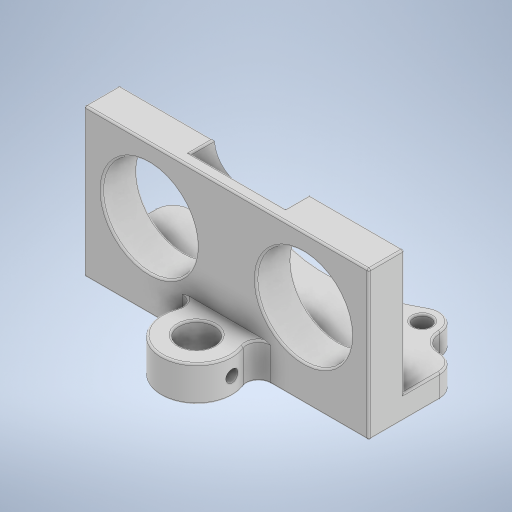
# Autodesk Inventor part: Front Sensor Mount
Saved by Autodesk Inventor 2023 (Build 270158000, 158)
## iProperties
Created: 2023-11-02
Part Number: Front Sensor Mount
Material: Generic
Document SubType Name: Modeling
Designer: Eric
Density: 1 g/cm^3
Appearance: Default
Author: Eric
Autodesk Inventor part; units mm, degrees
ref_plane "YZ Plane" through (0, 0, 0) normal (1, 0, 0) x (0, 1, 0)
ref_plane "XZ Plane" through (0, 0, 0) normal (0, 1, 0) x (-1, 0, 0)
ref_plane "XY Plane" through (0, 0, 0) normal (0, 0, 1) x (1, 0, 0)
sketch "Sketch1" plane through (0, 0, 0) normal (0, 1, 0) x (-1, 0, 0)
  circle A0 centre (15, -5) radius 1.45
  circle A1 centre (-15, -5) radius 1.45
  arc A2 (13.5033, -7.6) -> (18, -5) centre (15, -5) ccw
  arc A3 (-18, -5) -> (-13.5033, -7.6) centre (-15, -5) ccw
  arc A4 (13.5033, -7.6) -> (-13.5033, -7.6) centre (0, -31.058) ccw
  line L0 (24, 1) -> (24, 13)
  line L1 (-24, 1) -> (-24, 13)
  arc A5 (21, -2) -> (24, 1) centre (21, 1) ccw
  arc A6 (21, -2) -> (18, -5) centre (21, -5) ccw
  line L2 (0, -11.9168) -> (0, 19.826) construction
  arc A7 (-24, 1) -> (-21, -2) centre (-21, 1) ccw
  arc A8 (-18, -5) -> (-21, -2) centre (-21, -5) ccw
  circle A9 centre (0, 18) radius 3
  arc A10 (5.5621, 15.75) -> (-5.5621, 15.75) centre (0, 18) ccw
  line L3 (24, 13) -> (7.4162, 13)
  line L4 (-7.4162, 13) -> (-24, 13)
  arc A11 (5.5621, 15.75) -> (7.4162, 13) centre (7.4162, 15) ccw
  arc A12 (-7.4162, 13) -> (-5.5621, 15.75) centre (-7.4162, 15) ccw
  point P0 (0, 0)
  point P1 (0, 13)
  point P2 (3.3166, 13)
  point P3 (-3.3166, 13)
  dimension "d0" = 2.9
  dimension "d1" = 30
  dimension "d3" = 3
  dimension "d6" = 5
  dimension "d8" = 2.6
  dimension "d10" = 18
  dimension "d11" = 12
  dimension "d12" = 6
  dimension "d14" = 6
  dimension "d15" = 48
  dimension "d16" = 5
  dimension "d17" = 2
  constraints: 22 point on circle, 13 centre point, 12 end point, 9 tangent, 4 equal radius, 4 horizontal alignment, 4 symmetric about line, 3 concentric, 3 point on line, 3 vertical, 2 horizontal, 2 vertical alignment, 1 collinear, 2 other
  measures "d0" diameter of A0
  measures "d1" distance of A1.centre A0.centre
  measures "d3" radius of A2
  measures "d6" vertical distance of point (0, 0) A0.centre
  measures "d8" vertical distance of A0.centre A2.start
  measures "d10" vertical distance of A0.centre L0.end
  measures "d11" distance of L0.start L0.end
  measures "d12" diameter of A9
  measures "d14" radius of A10
  measures "d15" distance between parallel lines of L1 L0
  measures "d16" distance from line of L4 A9.centre
  measures "d17" radius of A11
extrude "Extrusion1" add sketch "Sketch1" along normal blind 4
sketch "Sketch3" plane through (0, 4, 0) normal (0, 1, 0) x (1, 0, 0)
  line L0 (-24, -13) -> (-7.4162, -13) projected
  line L1 (24, -13) -> (24, -1) projected
  line L2 (-24, -13) -> (24, -13)
  line L3 (24, -13) -> (24, -7)
  line L4 (24, -7) -> (-24, -7)
  line L5 (-24, -7) -> (-24, -13)
  point P0 (0, 0)
  dimension "d23" = 6
  constraints: 8 end point, 2 parallel, 1 horizontal, 1 midpoint, 1 perpendicular
  measures "d23" distance between parallel lines of L2 L4
extrude "Extrusion3" add sketch "Sketch3" along normal blind 21
sketch "Sketch4" plane through (7.4162, 0, 13) normal (0, 0, 1) x (1, 0, 0)
  circle A0 centre (-20.4162, 14) radius 8
  circle A1 centre (5.5838, 14) radius 8
  line L0 (-1.4162, 0) -> (-13.4162, 0) projected
  line L1 (-1.4162, 4) -> (-13.4162, 4) projected
  point P0 (-7.4162, 0)
  point P1 (-12.9783, 0)
  point P2 (-1.854, 0)
  point P3 (-7.4162, 0)
  point P4 (-12.9783, 4)
  point P5 (-1.854, 4)
  dimension "d26" = 26
  dimension "d27" = 16
  dimension "d28" = 13
  dimension "d29" = 10
  constraints: 2 centre point, 1 equal radius, 1 horizontal alignment, 1 midpoint
  measures "d26" distance of A1.centre A0.centre
  measures "d27" diameter of A1
  measures "d28" horizontal distance of point (-7.416, 0) A1.centre
  measures "d29" distance from line of L1 A1.centre
extrude "Extrusion4" cut sketch "Sketch4" against normal up to surface (6 mm away)
sketch "Sketch5" plane through (24, 4, 7) normal (0, 0, -1) x (-1, 0, 0)
  line L0 (18.5, 2.75) -> (29.5, 2.75) construction
  line L1 (20.75, 0.5) -> (27.25, 0.5)
  line L2 (27.25, 5) -> (20.75, 5)
  arc A0 (20.75, 5) -> (20.75, 0.5) centre (20.75, 2.75) ccw
  arc A1 (27.25, 0.5) -> (27.25, 5) centre (27.25, 2.75) ccw
  circle A2 centre (37, 10) radius 8 projected
  line L3 (48, 0) -> (0, 0) projected
  point P0 (24, -4)
  point P1 (24, 2.75)
  point P2 (18.5, 2.75)
  point P3 (24, 0)
  dimension "d32" = 11
  dimension "d33" = 4.5
  dimension "d34" = 9.5
  constraints: 8 end point, 7 point on circle, 4 tangent, 2 centre point, 2 midpoint, 2 point on line, 1 horizontal, 1 parallel, 1 vertical alignment
  measures "d32" distance of point (18.5, 2.75) L0.end
  measures "d33" distance between parallel lines of L1 L2
  measures "d34" distance from line of A2.centre L1
extrude "Extrusion5" cut sketch "Sketch5" against normal blind 4 contours A0 L2 A1 L1
sketch "Sketch6" plane through (24, 4, 7) normal (0, 0, -1) x (-1, 0, 0)
  line L0 (48, 21) -> (0, 21) projected
  line L1 (16, 21) -> (32, 21) construction
  line L2 (20.5, 25.5) -> (27.5, 25.5)
  line L3 (27.5, 16.5) -> (20.5, 16.5)
  arc A0 (20.5, 25.5) -> (20.5, 16.5) centre (20.5, 21) ccw
  arc A1 (27.5, 16.5) -> (27.5, 25.5) centre (27.5, 21) ccw
  line L4 (20.75, 5) -> (27.25, 5) projected
  point P0 (24, -4)
  point P1 (24, 21)
  point P2 (24, 5)
  point P3 (24, 5)
  point P4 (32, 21)
  point P5 (16, 21)
  dimension "d37" = 16
  dimension "d38" = 9
  constraints: 8 end point, 8 point on circle, 4 point on line, 4 tangent, 3 midpoint, 2 centre point, 1 parallel, 1 vertical alignment
  measures "d37" distance of point (16, 21) point (32, 21)
  measures "d38" distance between parallel lines of L2 L3
extrude "Extrusion6" cut sketch "Sketch6" against normal blind 4 contours A1 L3 A0 L0
sketch "Sketch7" plane through (0, 4, 0) normal (0, 1, 0) x (1, 0, 0)
  line L0 (7.4162, -13) -> (-7.4162, -13) projected
  arc A0 (7.4162, -13) -> (5.5621, -15.75) centre (7.4162, -15) ccw projected
  arc A1 (-5.5621, -15.75) -> (5.5621, -15.75) centre (0, -18) ccw projected
  arc A2 (-5.5621, -15.75) -> (-7.4162, -13) centre (-7.4162, -15) ccw projected
  circle A3 centre (0, -18) radius 3 projected
  point P0 (0, 0)
extrude "Extrusion7" add sketch "Sketch7" along normal blind 2
sketch "Sketch8" plane through (24, 0, 13) normal (1, 0, 0) x (0, 0, -1)
  line L0 (-8, 6) -> (-2, 6) projected
  circle A0 centre (-5, 3) radius 1.025
  point P0 (13, 0)
  point P1 (-5, 6)
  dimension "d43" = 2.05
  dimension "d44" = 3
  constraints: 1 centre point, 1 midpoint, 1 vertical alignment
  measures "d43" diameter of A0
  measures "d44" distance from line of L0 A0.centre
extrude "Extrusion8" cut sketch "Sketch8" against normal blind 24
fillet "Fillet1" radius 0.3 52 edges at (-24, 14.5, 7) (-24, 12.5, 13) (24, 12.5, 13) (24, 14.5, 7) (0, 25, 13) (24, 25, 10) (-24, 25, 10) (-16, 25, 7) (-8, 25, 9) (8, 25, 9) (16, 25, 7) (0, 25, 11) (0, 4.5, 7) (5.5, 6.75, 7) (0, 9, 7) (-5.5, 6.75, 7) (-21, 14, 7) (5, 14, 7) (5, 14, 13) (-21, 14, 13) (-3, 6, 18) (5.7579, 6, 13.882) (-5.7579, 6, 13.882) (0, 6, 24) (5.7579, 0, 13.882) (15.7081, 0, 13) (-5.7579, 0, 13.882) (-15.7081, 0, 13) (0, 0, 24) (3, 0, 18) (-16.5017, 4, -7.5971) (-18.8787, 4, -2.8787) (-23.1213, 4, -1.1213) (-24, 4, 4) (16.5017, 4, -7.5971) (18.8787, 4, -2.8787) (23.1213, 4, -1.1213) (24, 4, 4) (0, 4, -3.9911) (-16.5017, 0, -7.5971) (-18.8787, 0, -2.8787) (-23.1213, 0, -1.1213) (-24, 0, 7) (16.5017, 0, -7.5971) (18.8787, 0, -2.8787) (23.1213, 0, -1.1213) (24, 0, 7) (0, 0, -3.9911) (-13.55, 4, -5) (-13.55, 0, -5) (16.45, 4, -5) (16.45, 0, -5)
body "Solid1"
